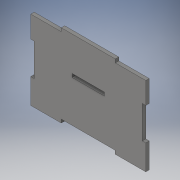
# Autodesk Inventor part: BASE_TAPAFIJA
Saved by Autodesk Inventor 2019 (Build 230136000, 136)
## iProperties
Created: 2020-02-12
Part Number: BASE_TAPAFIJA
Material: Genérico
Document SubType Name: Modeling
Designer: omar-
Density: 1 g/cm^3
Appearance: Valor por defecto
Author: omar-
Autodesk Inventor part; units mm, degrees
ref_plane "YZ Plane" through (0, 0, 0) normal (1, 0, 0) x (0, 1, 0)
ref_plane "XZ Plane" through (0, 0, 0) normal (0, 1, 0) x (-1, 0, 0)
ref_plane "XY Plane" through (0, 0, 0) normal (0, 0, 1) x (1, 0, 0)
sketch "Boceto1" plane through (0, 0, 0) normal (0, 0, 1) x (1, 0, 0)
  line L0 (-53.18, -36.59) -> (53.18, -36.59)
  line L1 (53.18, -36.59) -> (53.18, 36.59)
  line L2 (53.18, 36.59) -> (-53.18, 36.59)
  line L3 (-53.18, 36.59) -> (-53.18, -36.59)
  line L4 (-53.18, -36.59) -> (53.18, 36.59) construction
  line L5 (53.18, -36.59) -> (-53.18, 36.59) construction
  line L6 (-19.9778, -36.59) -> (30.0222, -36.59)
  line L7 (-25, 39.77) -> (25, 39.77)
  line L8 (25, 39.77) -> (25, 36.59)
  line L9 (25, 36.59) -> (-25, 36.59)
  line L10 (-25, 36.59) -> (-25, 39.77)
  line L11 (-53.18, 16.59) -> (-50, 16.59)
  line L12 (-50, 16.59) -> (-50, -13.41)
  line L13 (-50, -13.41) -> (-53.18, -13.41)
  line L14 (-53.18, -13.41) -> (-53.18, 16.59)
  line L15 (50, 16.59) -> (53.18, 16.59)
  line L16 (53.18, 16.59) -> (53.18, -13.41)
  line L17 (53.18, -13.41) -> (50, -13.41)
  line L18 (50, -13.41) -> (50, 16.59)
  line L19 (-25, -33.41) -> (25, -33.41)
  line L20 (25, -33.41) -> (25, -36.59)
  line L21 (25, -36.59) -> (-25, -36.59)
  line L22 (-25, -36.59) -> (-25, -33.41)
  line L23 (-15, 5) -> (15, 5)
  line L24 (15, 5) -> (15, 8.18)
  line L25 (15, 8.18) -> (-15, 8.18)
  line L26 (-15, 8.18) -> (-15, 5)
  line L27 (-15, 5) -> (15, 8.18) construction
  line L28 (15, 5) -> (-15, 8.18) construction
  point P0 (0, 0)
  point P1 (0, 6.59)
  dimension "d0" = 106.36
  dimension "d3" = 73.18
  dimension "d4" = 3.18
  dimension "d5" = 50
  dimension "d6" = 25
  dimension "d8" = 30
  dimension "d9" = 30
  dimension "d10" = 3.18
  dimension "d11" = 20
  dimension "d12" = 20
  dimension "d13" = 50
  dimension "d14" = 25
  dimension "d17" = 30
  dimension "d18" = 3.18
  dimension "d19" = 40
  dimension "d20" = 15
  constraints: 58 end point, 12 parallel, 7 horizontal, 6 perpendicular, 5 collinear, 4 midpoint, 2 equal length
  measures "d0" distance of L2.end L1.end
  measures "d3" distance of L0.end L1.end
  measures "d4" distance of L7.end L8.end
  measures "d5" distance of L7.start L7.end
  measures "d6" distance from line of point (0, 0) L8
  measures "d8" distance of L11.end L12.end
  measures "d9" distance of L17.end L15.start
  measures "d10" distance of L15.start L15.end
  measures "d11" distance between parallel lines of L2 L15
  measures "d12" distance between parallel lines of L2 L11
  measures "d13" distance of L19.start L19.end
  measures "d14" distance from line of L20 point (0, 0)
  measures "d17" distance of L25.end L24.end
  measures "d18" distance of L24.end L23.end
  measures "d19" distance from line of L19 point (0, 6.59)
  measures "d20" distance from line of point (0, 0) L24
extrude "Extrusión1" add sketch "Boceto1" along normal blind 3.18 contours L3 L13 L12 L11 L2 L1 L15 L18 L17 L0 L20 L19 L22 | L10 L7 L8 L2
